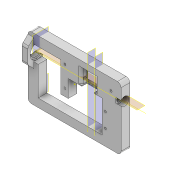
# Autodesk Inventor part: 10_Wellplate_base_v3
Saved by Autodesk Inventor 2022 (Build 260153000, 153)
## iProperties
Created: 2022-04-18
Part Number: 10_Wellplate_base_v3
Material: Generic
Document SubType Name: Modeling
Designer: Prakash Lab
Density: 1 g/cm^3
Appearance: Default
Author: Prakash Lab
Autodesk Inventor part; units mm, degrees
ref_plane "YZ Plane" through (0, 0, 0) normal (1, 0, 0) x (0, 1, 0)
ref_plane "XZ Plane" through (0, 0, 0) normal (0, 1, 0) x (-1, 0, 0)
ref_plane "XY Plane" through (0, 0, 0) normal (0, 0, 1) x (1, 0, 0)
sketch "Sketch1" plane through (0, 0, 0) normal (0, 0, 1) x (1, 0, 0)
  line L0 (63.9, -42.75) -> (-63.9, -42.75)
  line L1 (-63.9, -42.75) -> (-63.9, 42.75)
  line L2 (-63.9, 42.75) -> (63.9, 42.75)
  line L3 (63.9, 42.75) -> (63.9, -42.75)
  line L4 (63.9, -42.75) -> (-63.9, 42.75) construction
  line L5 (-63.9, -42.75) -> (63.9, 42.75) construction
  point P0 (0, 0)
  dimension "d0" = 127.8
  dimension "d1" = 85.5
  constraints: 12 end point, 2 midpoint, 2 parallel, 1 horizontal, 1 perpendicular
  measures "d0" distance of L0.start L0.end
  measures "d1" distance of L0.end L1.end
extrude "Extrusion1" add sketch "Sketch1" along normal blind 12
fillet "Fillet1" radius 4 4 edges at (63.9, 42.75, 6) (-63.9, 42.75, 6) (-63.9, -42.75, 6) (63.9, -42.75, 6)
sketch "Sketch2" plane through (0, 0, 12) normal (0, 0, 1) x (1, 0, 0)
  arc A0 (59.9, -42.75) -> (63.9, -38.75) centre (59.9, -38.75) ccw projected
  line L0 (63.9, -38.75) -> (63.9, 38.75) projected
  arc A1 (63.9, 38.75) -> (59.9, 42.75) centre (59.9, 38.75) ccw projected
  line L1 (59.9, 42.75) -> (-59.9, 42.75) projected
  arc A2 (-59.9, 42.75) -> (-63.9, 38.75) centre (-59.9, 38.75) ccw projected
  line L2 (-63.9, 38.75) -> (-63.9, -38.75) projected
  arc A3 (-63.9, -38.75) -> (-59.9, -42.75) centre (-59.9, -38.75) ccw projected
  line L3 (-59.9, -42.75) -> (59.9, -42.75) projected
  line L4 (28, 3) -> (9, 3)
  line L5 (9, 3) -> (9, 22)
  line L6 (9, 22) -> (28, 22)
  line L7 (28, 22) -> (28, 3)
  line L8 (28, 3) -> (9, 22) construction
  line L9 (9, 3) -> (28, 22) construction
  line L10 (18.6, 3.8849) -> (18.6, 4.1649)
  point P0 (0, 0)
  point P1 (18.5, 12.5)
  dimension "d5" = 19
  dimension "d6" = 19
  dimension "d221" = 3
  dimension "d223" = 18.5
  constraints: 14 end point, 2 midpoint, 2 parallel, 1 horizontal, 1 perpendicular, 1 vertical, 2 other
  measures "d5" distance of L5.end L6.end
  measures "d6" distance of L4.end L5.end
  measures "d221" vertical distance of L4.end point (0, 0)
  measures "d223" horizontal distance of point (0, 0) point (18.5, 12.5)
extrude "Extrusion2" cut sketch "Sketch2" against normal blind 8 contours L4 L5 L6 L7
sketch "Sketch3" plane through (0, 0, 4) normal (0, 0, 1) x (1, 0, 0)
  line L0 (9, 22) -> (28, 22) projected
  line L1 (9, 3) -> (9, 22) projected
  line L2 (28, 3) -> (9, 3) projected
  line L3 (28, 22) -> (28, 3) projected
  line L4 (26.5, 20.5) -> (10.5, 20.5)
  line L5 (10.5, 20.5) -> (10.5, 4.5)
  line L6 (10.5, 4.5) -> (26.5, 4.5)
  line L7 (26.5, 4.5) -> (26.5, 20.5)
  point P0 (0, 0)
  dimension "d11" = 1.5
  constraints: 8 end point, 3 other
  measures "d11" distance between parallel lines of L0 L4
extrude "Extrusion3" cut sketch "Sketch3" against normal through all contours L7 L6 L5 L4
ref_plane "Work Plane1" through (18.5, 3, 12) normal (-1, 0, 0) x (0, 0, 1)
ref_plane "Work Plane2" through (9, 12.5, 12) normal (0, 1, 0) x (1, 0, 0)
chamfer "Chamfer1" distance 4 angle 45 4 edges at (18.5, 4.5, 0) (26.5, 12.5, 0) (18.5, 20.5, 0) (10.5, 12.5, 0)
ref_plane "Work Plane3" through (28.5, 3, 12) normal (-1, 0, 0) x (0, 0, 1)
sketch "Sketch12" plane through (63.9, -38.75, 0) normal (1, 0, 0) x (0, 0, -1)
  circle A0 centre (-7.125, 48) radius 4.2 construction
  circle A1 centre (-7.125, 48) radius 4.5
  point P0 (0, 38.75)
  dimension "d100" = 9
  constraints: 1 centre point
  measures "d100" diameter of A1
extrude "Extrusion12" cut sketch "Sketch12" against normal up to surface (35.9 mm away) draft -4
sketch "Sketch13" plane through (63.9, -38.75, 0) normal (1, 0, 0) x (0, 0, -1)
  arc A0 (-10, 44.9382) -> (-10, 51.0618) centre (-7.125, 48) ccw projected
  circle A1 centre (-7.125, 48) radius 6
  point P0 (0, 38.75)
  dimension "d63" = 12
  constraints: 1 centre point, 1 coincident
  measures "d63" diameter of A1
extrude "Extrusion13" cut sketch "Sketch13" against normal blind 7
mirror "Mirror1" about plane through (18.5, 3, 12) normal (-1, 0, 0) of "Extrusion12", "Extrusion13"
ref_plane "Work Plane4" through (-47.9, 27.75, 11) normal (-1, 0, 0) x (0, 0, 1)
ref_plane "Work Plane5" through (-39.7, 19.25, 21) normal (0, 0, 1) x (1, 0, 0)
ref_plane "Arbeitsebene7" through (-58.9, -38.75, 0) normal (-1, 0, 0) x (0, 0, 1)
sketch "Skizze28" plane through (-58.9, -38.75, 0) normal (-1, 0, 0) x (0, 0, 1)
  line L0 (17.125, 56.5) -> (17.125, 39.5) projected
  arc A0 (17.125, 56.5) -> (15.625, 58) centre (15.625, 56.5) ccw projected
  line L1 (-1.375, 58) -> (15.625, 58) projected
  arc A1 (-1.375, 58) -> (-2.875, 56.5) centre (-1.375, 56.5) ccw projected
  line L2 (-2.875, 39.5) -> (-2.875, 56.5) projected
  arc A2 (-2.875, 39.5) -> (-1.375, 38) centre (-1.375, 39.5) ccw projected
  line L3 (15.625, 38) -> (-1.375, 38) projected
  arc A3 (15.625, 38) -> (17.125, 39.5) centre (15.625, 39.5) ccw projected
  circle A4 centre (15.125, 56) radius 0.7835 projected
  circle A5 centre (15.125, 40) radius 0.7835 projected
  circle A6 centre (-0.875, 56) radius 0.7835 projected
  circle A7 centre (-0.875, 40) radius 0.7835 projected
  circle A8 centre (7.125, 48) radius 7.5 projected
  arc A9 (17.625, 56.5) -> (15.625, 58.5) centre (15.625, 56.5) ccw
  line L4 (17.625, 56.5) -> (17.625, 39.5)
  arc A10 (15.625, 37.5) -> (17.625, 39.5) centre (15.625, 39.5) ccw
  line L5 (15.625, 37.5) -> (-1.375, 37.5)
  arc A11 (-3.375, 39.5) -> (-1.375, 37.5) centre (-1.375, 39.5) ccw
  line L6 (-3.375, 39.5) -> (-3.375, 56.5)
  arc A12 (-1.375, 58.5) -> (-3.375, 56.5) centre (-1.375, 56.5) ccw
  line L7 (-1.375, 58.5) -> (15.625, 58.5)
  point P0 (0, 38.75)
  dimension "d142" = 0.5
  constraints: 8 end point, 8 point on circle, 4 centre point, 7 other
  measures "d142" distance between parallel lines of L1 L7
extrude "Extrusion27" cut sketch "Skizze28" against normal blind 40 contours L0 A3 L3 A2 L2 A1 L1 A0 | A4 | A5 | A6 | A7 | A8 | L4 A10 L5 A11 L6 A12 L7 A9
sketch "Skizze29" plane through (-63.9, -38.75, 0) normal (-1, 0, 0) x (0, 0, 1)
  line L0 (17.125, 56.5) -> (17.125, 39.5) projected
  arc A0 (17.125, 56.5) -> (15.625, 58) centre (15.625, 56.5) ccw projected
  line L1 (-1.375, 58) -> (15.625, 58) projected
  arc A1 (-1.375, 58) -> (-2.875, 56.5) centre (-1.375, 56.5) ccw projected
  line L2 (-2.875, 39.5) -> (-2.875, 56.5) projected
  arc A2 (-2.875, 39.5) -> (-1.375, 38) centre (-1.375, 39.5) ccw projected
  line L3 (15.625, 38) -> (-1.375, 38) projected
  arc A3 (15.625, 38) -> (17.125, 39.5) centre (15.625, 39.5) ccw projected
  circle A4 centre (15.125, 56) radius 0.7835 projected
  circle A5 centre (15.125, 40) radius 0.7835 projected
  circle A6 centre (-0.875, 56) radius 0.7835 projected
  circle A7 centre (-0.875, 40) radius 0.7835 projected
  circle A8 centre (7.125, 48) radius 7.5 projected
  line L4 (0, 77.5) -> (0, 0) projected
  line L5 (12, 77.5) -> (12, 0) projected
  line L6 (12, 0) -> (12, 44.5022) projected
  line L7 (12, 29.511) -> (18.807, 36.318)
  line L8 (18.807, 59.682) -> (10, 68.489)
  line L9 (10, 68.5) -> (10, 31.5) projected
  line L10 (20.125, 39.5) -> (20.125, 56.5)
  arc A9 (20.125, 56.5) -> (15.625, 61) centre (15.625, 56.5) ccw
  line L11 (15.625, 61) -> (-1.375, 61)
  arc A10 (-1.375, 61) -> (-5.875, 56.5) centre (-1.375, 56.5) ccw
  line L12 (-5.875, 56.5) -> (-5.875, 39.5)
  arc A11 (-5.875, 39.5) -> (-1.375, 35) centre (-1.375, 39.5) ccw
  line L13 (-1.375, 35) -> (15.625, 35)
  arc A12 (15.625, 35) -> (20.125, 39.5) centre (15.625, 39.5) ccw
  point P0 (0, 38.75)
  point P1 (0, 58)
  point P2 (0, 38)
  point P3 (10, 11.9077)
  point P4 (10, 31.5)
  point P5 (12, 38)
  point P6 (12, 66.489)
  point P7 (12, 58)
  point P8 (10, 10.3787)
  point P9 (0, 45.6581)
  point P10 (0, 50.3419)
  dimension "d151" = 45
  dimension "d152" = 45
  dimension "d224" = 3
  constraints: 12 end point, 10 point on circle, 4 centre point, 1 tangent, 12 other
  measures "d151" angle of L1 L8
  measures "d152" angle of L3 L7
  measures "d224" distance between parallel lines of L0 L10
extrude "Extrusion28" add sketch "Skizze29" against normal blind 8 contours A0 L1 L5 L11 A9 L10 A12 L13 L3 A3 L0 | L0 A3 L3 L5 A8 L1 A0 | L5 A8 L9 L1 | L3 L9 A8 L5 | L9 A8 L4 L1 | L5 L8 A9 L11 | L3 L4 A8 L9 | L13 A12 L7 L5 | L4 A8 | A4 | A5
sketch "Skizze30" plane through (-55.9, -38.75, 0) normal (1, 0, 0) x (0, 0, -1)
  circle A0 centre (-7.125, 48) radius 7.3 projected
  circle A1 centre (-7.125, 48) radius 7.8
  point P0 (0, 38.75)
  dimension "d147" = 0.5
  constraints: 1 centre point
  measures "d147" radial gap between concentric circles of A0 A1
extrude "Extrusion29" cut sketch "Skizze30" against normal up to surface (8 mm away) contours A0 | A1
fillet "Rundung6" radius 2 2 edges at (-59.9, 6.076, 0) (-59.9, 12.424, 0)
sketch "Skizze40" plane through (0, 0, 12) normal (0, 0, 1) x (1, 0, 0)
  line L0 (-63.9, -9.239) -> (-63.9, -38.75) projected
  arc A0 (-63.9, -38.75) -> (-59.9, -42.75) centre (-59.9, -38.75) ccw projected
  line L1 (-59.9, -42.75) -> (59.9, -42.75) projected
  arc A1 (59.9, -42.75) -> (63.9, -38.75) centre (59.9, -38.75) ccw projected
  line L2 (63.9, -38.75) -> (63.9, 5.7522) projected
  line L3 (63.9, 5.7522) -> (56.9, 5.7522) projected
  line L4 (56.9, 5.7522) -> (56.9, 12.7478) projected
  line L5 (56.9, 12.7478) -> (63.9, 12.7478) projected
  line L6 (63.9, 12.7478) -> (63.9, 38.75) projected
  arc A2 (63.9, 38.75) -> (59.9, 42.75) centre (59.9, 38.75) ccw projected
  line L7 (59.9, 42.75) -> (-59.9, 42.75) projected
  arc A3 (-59.9, 42.75) -> (-63.9, 38.75) centre (-59.9, 38.75) ccw projected
  line L8 (-63.9, 38.75) -> (-63.9, 27.739) projected
  line L9 (-55.9, 19.75) -> (-18.9, 19.75) projected
  line L10 (-18.9, 19.75) -> (-18.9, -1.25) projected
  line L11 (-18.9, -1.25) -> (-55.9, -1.25) projected
  line L12 (63.9, 12.7478) -> (63.9, 38.75) projected
  line L13 (-63.9, 42.75) -> (63.9, 42.75)
  line L14 (63.9, 42.75) -> (63.9, 32.75)
  line L15 (63.9, 32.75) -> (-63.9, 32.75)
  line L16 (-63.9, 32.75) -> (-63.9, 42.75)
  line L17 (-55.9, 27.739) -> (-55.9, 19.75) projected
  line L18 (-55.9, -1.25) -> (-55.9, -9.239) projected
  line L19 (-55.9, -9.239) -> (-63.9, -9.239) projected
  line L20 (-63.9, 27.739) -> (-55.9, 27.739) projected
  point P0 (0, 0)
  point P1 (-59.9, 42.75)
  dimension "d178" = 10
  constraints: 8 end point, 2 parallel, 1 horizontal, 1 perpendicular, 1 point on line
  measures "d178" distance of L13.end L14.end
extrude "Extrusion37" cut sketch "Skizze40" against normal through all contours L8 A3 L7 A2 L6 L15 | L16 L13 A3 | A2 L13 L14
sketch "Skizze41" plane through (0, 0, 12) normal (0, 0, 1) x (1, 0, 0)
  line L0 (63.9, 32.75) -> (-63.9, 32.75) projected
  line L1 (-63.9, 32.75) -> (-63.9, 27.739) projected
  line L2 (-55.9, 19.75) -> (-18.9, 19.75) projected
  line L3 (-18.9, 19.75) -> (-18.9, -1.25) projected
  line L4 (-18.9, -1.25) -> (-55.9, -1.25) projected
  line L5 (-63.9, -9.239) -> (-63.9, -38.75) projected
  arc A0 (-63.9, -38.75) -> (-59.9, -42.75) centre (-59.9, -38.75) ccw projected
  line L6 (-59.9, -42.75) -> (59.9, -42.75) projected
  arc A1 (59.9, -42.75) -> (63.9, -38.75) centre (59.9, -38.75) ccw projected
  line L7 (63.9, -38.75) -> (63.9, 5.7522) projected
  line L8 (63.9, 5.7522) -> (56.9, 5.7522) projected
  line L9 (56.9, 5.7522) -> (56.9, 12.7478) projected
  line L10 (56.9, 12.7478) -> (63.9, 12.7478) projected
  line L11 (63.9, 12.7478) -> (63.9, 32.75) projected
  line L12 (-63.9, -38.75) -> (63.9, -38.75)
  line L13 (63.9, -38.75) -> (63.9, -52.75)
  line L14 (63.9, -52.75) -> (-63.9, -52.75)
  line L15 (-63.9, -52.75) -> (-63.9, -38.75)
  line L16 (-63.9, 27.739) -> (-55.9, 27.739) projected
  line L17 (-55.9, 27.739) -> (-55.9, 19.75) projected
  line L18 (-55.9, -1.25) -> (-55.9, -9.239) projected
  line L19 (-55.9, -9.239) -> (-63.9, -9.239) projected
  point P0 (0, 0)
  dimension "d181" = 14
  constraints: 8 end point, 2 parallel, 1 horizontal, 1 perpendicular
  measures "d181" distance of L12.end L13.end
extrude "Extrusion38" add sketch "Skizze41" against normal up to surface (12 mm away) contours L13 L14 L15 A0 L6 A1
fillet "Rundung7" radius 5 4 edges at (-63.9, 32.75, 6) (63.9, 32.75, 6) (-63.9, -52.75, 6) (63.9, -52.75, 6)
sketch "Skizze42" plane through (0, 0, 12) normal (0, 0, 1) x (1, 0, 0)
  line L0 (34.4, -33.4236) -> (34.4, -16.1764)
  arc A0 (30.4, -33.4236) -> (34.4, -33.4236) centre (32.4, -33.4236) ccw
  line L1 (30.4, -16.1764) -> (30.4, -33.4236)
  arc A1 (34.4, -16.1764) -> (30.4, -16.1764) centre (32.4, -16.1764) ccw
  line L2 (25.4, -33.4236) -> (25.4, -21.25)
  arc A2 (25.4, -33.4236) -> (25.7804, -35.6997) centre (32.4, -33.4236) ccw
  arc A3 (23.8891, -38.35) -> (25.7804, -35.6997) centre (23.8891, -36.35) ccw
  line L3 (37.373, -38.35) -> (23.8891, -38.35)
  arc A4 (37.373, -38.35) -> (37.4, -38.3226) centre (32.4, -33.4236) ccw
  line L4 (37.4, -11.2774) -> (37.4, -38.3226)
  arc A5 (37.4, -11.2774) -> (37.373, -11.25) centre (32.4, -16.1764) ccw
  line L5 (27.427, -11.25) -> (37.373, -11.25)
  arc A6 (27.427, -11.25) -> (27.4, -11.2774) centre (32.4, -16.1764) ccw
  line L6 (27.4, -19.25) -> (27.4, -11.2774)
  arc A7 (25.4, -21.25) -> (27.4, -19.25) centre (25.4, -19.25) ccw
  arc A8 (12.0825, -21.5243) -> (11.6348, -21.331) centre (11.0716, -23.25) ccw
  spline S0 degree 3 poles (12.0825, -21.5243) (11.8555, -21.3913) (11.6488, -21.229) (11.2907, -20.8371) (11.1452, -20.6102) (10.9547, -20.1287) (10.906, -19.8824) (10.906, -19.633) knots 0 0 0 0 0.335568 0.335568 0.679419 0.679419 1 1 1 1
  line L7 (10.906, -11.25) -> (10.906, -19.633)
  line L8 (-7.9188, -11.25) -> (10.906, -11.25)
  arc A9 (-7.9188, -11.25) -> (-8.1, -11.4342) centre (-3.0199, -16.25) ccw
  line L9 (-8.1, -21.0658) -> (-8.1, -11.4342)
  arc A10 (-8.1, -21.0658) -> (-3.0199, -23.25) centre (-3.0199, -16.25) ccw
  line L10 (6.8199, -23.25) -> (-3.0199, -23.25)
  arc A11 (6.8199, -23.25) -> (11.6348, -21.331) centre (6.8199, -16.25) ccw
  arc A12 (-3.0199, -14.25) -> (-3.0199, -18.25) centre (-3.0199, -16.25) ccw
  line L11 (6.8199, -14.25) -> (-3.0199, -14.25)
  arc A13 (6.8199, -18.25) -> (6.8199, -14.25) centre (6.8199, -16.25) ccw
  line L12 (-3.0199, -18.25) -> (6.8199, -18.25)
  line L13 (11.7188, -21.25) -> (25.4, -21.25)
  arc A14 (6.8199, -23.25) -> (11.7188, -21.25) centre (6.8199, -16.25) ccw
  line L14 (6.8199, -23.25) -> (-3.0199, -23.25)
  arc A15 (-8.1, -21.0658) -> (-3.0199, -23.25) centre (-3.0199, -16.25) ccw
  line L15 (-8.1, -38.35) -> (-8.1, -21.0658)
  line L16 (2.9, -38.35) -> (-8.1, -38.35)
  line L17 (2.9, -32.85) -> (2.9, -38.35)
  line L18 (22.3, -32.85) -> (2.9, -32.85)
  line L19 (22.3, -32.85) -> (22.3, -38.35)
  line L20 (22.3, -38.35) -> (23.8891, -38.35)
  arc A16 (23.8891, -38.35) -> (25.7804, -35.6997) centre (23.8891, -36.35) ccw
  arc A17 (25.4, -33.4236) -> (25.7804, -35.6997) centre (32.4, -33.4236) ccw
  line L21 (25.4, -33.4236) -> (25.4, -21.25)
  circle A18 centre (6.8199, -6.25) radius 3.25
  circle A19 centre (32.4, -6.25) radius 3.25
  circle A20 centre (-3.0199, -6.25) radius 3.25
  line L22 (-18.1, -1.25) -> (47.4, -1.25)
  line L23 (-58.9, -52.75) -> (58.9, -52.75)
  line L24 (58.9, -52.75) -> (-58.9, -52.75)
  line L25 (7.9, -11.25) -> (27.427, -11.25)
  line L26 (47.4, -11.25) -> (47.4, -1.25)
  line L27 (-18.1, -1.25) -> (-18.1, -21.25)
  line L28 (-11.5, -4.75) -> (-11.5, -17.75)
  arc A21 (-14.7, -17.75) -> (-11.5, -17.75) centre (-13.1, -17.75) ccw
  line L29 (-14.7, -17.75) -> (-14.7, -4.75)
  arc A22 (-11.5, -4.75) -> (-14.7, -4.75) centre (-13.1, -4.75) ccw
  line L30 (43.973, -4.75) -> (43.973, -17.75)
  arc A23 (40.773, -17.75) -> (43.973, -17.75) centre (42.373, -17.75) ccw
  line L31 (40.773, -17.75) -> (40.773, -4.75)
  arc A24 (43.973, -4.75) -> (40.773, -4.75) centre (42.373, -4.75) ccw
  line L32 (47.373, -11.25) -> (47.4, -11.25)
  line L33 (27.4, -11.2774) -> (27.4, -21.25)
  line L34 (27.4, -21.25) -> (37.4, -21.25)
  line L35 (-18.1, -21.25) -> (7.9, -21.25)
  line L36 (7.9, -21.25) -> (7.9, -11.25)
  line L37 (40.7865, -37.3611) -> (40.7865, -24.3611)
  arc A25 (43.9865, -24.3611) -> (40.7865, -24.3611) centre (42.3865, -24.3611) ccw
  line L38 (43.9865, -24.3611) -> (43.9865, -37.3611)
  arc A26 (40.7865, -37.3611) -> (43.9865, -37.3611) centre (42.3865, -37.3611) ccw
  line L39 (37.4, -21.25) -> (37.4, -41.25)
  line L40 (37.4, -41.25) -> (47.373, -41.25)
  line L41 (47.373, -41.25) -> (47.373, -11.25)
  line L42 (-58.9, -1.25) -> (-18.9, -1.25)
  line L43 (-49.9, -1.25) -> (-8.6, -1.25)
  line L44 (-8.6, -1.25) -> (-8.6, -41.35)
  line L45 (-8.6, -41.35) -> (-49.9, -41.35)
  line L46 (-49.9, -41.35) -> (-49.9, -1.25)
  line L47 (-63.9, -9.239) -> (-63.9, -47.75)
  line L48 (26.5, 4.5) -> (10.5, 4.5)
  line L49 (-8.6, 3.5) -> (37.9, 3.5)
  line L50 (37.9, 3.5) -> (37.9, -41.35)
  line L51 (37.9, -41.35) -> (-8.6, -41.35)
  line L52 (-8.6, -41.35) -> (-8.6, 3.5)
  circle A27 centre (-13.1, -11.2637) radius 1.4
  circle A28 centre (42.4, -11.2637) radius 1.4
  circle A29 centre (42.4, -31.25) radius 1.4
  line L53 (-18.9, 19.75) -> (-18.9, -1.25)
  line L54 (-18.1, -1.25) -> (-18.9, -1.25)
  line L55 (-18.9, -1.25) -> (-18.9, -21.25)
  line L56 (-18.9, -21.25) -> (-18.1, -21.25)
  line L57 (-18.1, -21.25) -> (-18.1, -1.25)
  arc A30 (27.427, -11.25) -> (27.4, -11.2774) centre (32.4, -16.1764) ccw
  line L58 (-18.9, -21.25) -> (-8.6, -21.25)
  line L59 (-8.6, -21.25) -> (-8.6, -41.35)
  line L60 (-8.6, -41.35) -> (-18.9, -41.35)
  line L61 (-18.9, -41.35) -> (-18.9, -21.25)
  point P0 (37.4, -13.25)
  point P1 (47.373, -21.25)
  point P2 (-8.1, -21.25)
  point P3 (-8.6, -38.75)
  point P4 (-8.6, -21.25)
  point P5 (-18.9, 10.3274)
  point P6 (-8.6, -21.25)
  point P7 (-63.9, -0.75)
  dimension "d199" = 14
  dimension "d201" = 0.5
  dimension "d203" = 0.5
  dimension "d204" = 1
  dimension "d205" = 3
  dimension "d206" = 2.8
  dimension "d207" = 2.8
  dimension "d208" = 2.8
  constraints: 32 end point, 8 parallel, 4 horizontal, 4 perpendicular, 3 centre point, 2 point on line, 1 other
  measures "d199" distance between parallel lines of L47 L46
  measures "d201" distance from line of L9.end L52
  measures "d203" distance between parallel lines of L4 L50
  measures "d204" distance between parallel lines of L48 L49
  measures "d205" distance between parallel lines of L3 L51
  measures "d206" diameter of A27
  measures "d207" diameter of A28
  measures "d208" diameter of A29
extrude "Extrusion39" cut sketch "Skizze42" against normal through all contours A0 L1 L34 L0 | L0 L34 L4 A4 L3 A3 A2 L2 A7 L33 L1 A0 | L34 L1 A1 L0 | L0 A1 L1 L34 L33 L6 A6 L5 A5 L4 | L4 A5 L5 L25 L8 A9 L9 L15 L35 L44 L22 L50 L40 L39 | L39 L40 L50 L51 L44 L35 L15 L16 L17 L18 L19 L20 L3 A4 | A7 L13 A14 S0 L7 L25 A6 L6 | L2 A2 A3 L20 L19 L18 L17 L16 L15 L35 A10 L10 A11 A8 S0 A14 L13 | L7 S0 A14 A11 L10 A10 L35 L36 A13 L8 | L22 L52 L49 L50 | S0 A8 A14 | L36 A13 L11 A12 L12 L35 A10 L9 A9 L8 | L45 L61 L56 L35 L44 | L36 A13 L12 A12 L11 | A13 L36 | L45 L46 L42 L55 L61 | L15 A10 L35 | A18 | A19 | A20 | A27 | A28 | A29
sketch "Skizze44" plane through (0, 0, 12) normal (0, 0, 1) x (1, 0, 0)
  point P0 (0, 0)
sketch "Skizze45" plane through (-55.9, -38.75, 0) normal (1, 0, 0) x (0, 0, -1)
  arc A0 (-3.0459, 54.6484) -> (-3.0459, 41.3516) centre (-7.125, 48) ccw projected
  circle A1 centre (-7.125, 48) radius 10
  point P0 (0, 38.75)
  dimension "d195" = 20
  constraints: 1 centre point, 1 coincident
  measures "d195" diameter of A1
extrude "Extrusion41" cut sketch "Skizze45" against normal blind 2
sketch "Skizze46" plane through (0, 0, 12) normal (0, 0, 1) x (1, 0, 0)
  line L0 (-8.6, 3.5) -> (9, 3.5) projected
  line L1 (9, 3.5) -> (9, 22) projected
  line L2 (9, 22) -> (28, 22) projected
  line L3 (28, 22) -> (28, 3.5) projected
  line L4 (37.9, 3.5) -> (37.9, -41.35) projected
  line L5 (37.9, -41.35) -> (-49.9, -41.35) projected
  line L6 (-49.9, -41.35) -> (-49.9, -1.25) projected
  line L7 (-49.9, -1.25) -> (-55.9, -1.25) projected
  line L8 (-63.9, -9.239) -> (-63.9, -47.75) projected
  arc A0 (-63.9, -47.75) -> (-58.9, -52.75) centre (-58.9, -47.75) ccw projected
  line L9 (-58.9, -52.75) -> (58.9, -52.75) projected
  arc A1 (58.9, -52.75) -> (63.9, -47.75) centre (58.9, -47.75) ccw projected
  line L10 (63.9, -47.75) -> (63.9, 5.7522) projected
  line L11 (63.9, 5.7522) -> (56.9, 5.7522) projected
  line L12 (56.9, 5.7522) -> (56.9, 12.7478) projected
  line L13 (56.9, 12.7478) -> (63.9, 12.7478) projected
  line L14 (63.9, 12.7478) -> (63.9, 27.75) projected
  arc A2 (63.9, 27.75) -> (58.9, 32.75) centre (58.9, 27.75) ccw projected
  line L15 (58.9, 32.75) -> (-58.9, 32.75) projected
  arc A3 (-58.9, 32.75) -> (-63.9, 27.75) centre (-58.9, 27.75) ccw projected
  line L16 (-55.9, 19.75) -> (-18.9, 19.75) projected
  line L17 (-18.9, 19.75) -> (-18.9, -21.25) projected
  line L18 (-18.9, -21.25) -> (-8.6, -21.25) projected
  line L19 (-8.6, -21.25) -> (-8.6, 3.5) projected
  circle A4 centre (42.4, -31.25) radius 1.4 projected
  circle A5 centre (42.4, -11.2637) radius 1.4 projected
  circle A6 centre (-13.1, -11.2637) radius 1.4 projected
  circle A7 centre (-13.1, 17.25) radius 1.4
  circle A8 centre (50.2191, 17.25) radius 1.4
  line L20 (28, 3.5) -> (37.9, 3.5) projected
  line L21 (-55.9, -1.25) -> (-55.9, -9.239) projected
  line L22 (-55.9, -9.239) -> (-63.9, -9.239) projected
  line L23 (-63.9, 27.739) -> (-55.9, 27.739) projected
  line L24 (-55.9, 27.739) -> (-55.9, 19.75) projected
  line L25 (-63.9, 27.75) -> (-63.9, 27.739) projected
  point P0 (0, 0)
  dimension "d209" = 2.8
  dimension "d210" = 2.8
  constraints: 2 centre point
  measures "d209" diameter of A7
  measures "d210" diameter of A8
extrude "Extrusion42" cut sketch "Skizze46" against normal through all contours A7 | A8
sketch "Skizze49" plane through (0, 0, 0) normal (0, 0, -1) x (-1, 0, 0)
  line L0 (9.6, 5.25) -> (2.6, 5.25) projected
  line L1 (-26.5, 4.5) -> (-10.5, 4.5) projected
  line L2 (6.6, 5.45) -> (-43.4, 5.45) projected
  line L3 (-37.9, 2.25) -> (-37.9, 5.25) projected
  line L4 (-30.5, 24.5) -> (-30.5, 3.5) projected
  line L5 (8.6, 2.25) -> (9.6, 2.25) projected
  line L6 (-46.4, 2.25) -> (-37.9, 2.25)
  line L7 (-37.9, 2.25) -> (-37.9, 4.5)
  line L8 (-37.9, 4.5) -> (-46.4, 4.5)
  line L9 (-46.4, 4.5) -> (-46.4, 2.25)
  line L10 (8.6, 2.25) -> (9.6, 2.25) projected
  line L11 (-37.9, 4.5) -> (9.6, 4.5)
  line L12 (9.6, 4.5) -> (9.6, 2.25)
  line L13 (9.6, 2.25) -> (-37.9, 2.25)
  line L14 (-37.9, 2.25) -> (-37.9, 4.5)
  point P0 (0, 0)
  point P1 (8.6, 2.25)
  point P2 (-10.5, 4.5)
  point P3 (-42.4, 6.25)
  point P4 (-41.0667, 6.25)
  point P5 (-30.5, 3.5)
  constraints: 16 end point, 4 parallel, 2 horizontal, 2 perpendicular, 1 point on line, 1 other
ref_plane "Arbeitsebene10" through (-6.6, 5.45, 2.125) normal (0, 0, -1) x (0, 1, 0)
extrude "Extrusion45" add sketch "Skizze49" against normal up to surface (4 mm away) contours L3 L6 L9 L8
sketch "Skizze50" plane through (-8.6, 3.5, 12) normal (0, -1, 0) x (1, 0, 0)
  line L0 (17.6, 0) -> (36.6, 0) projected
  line L1 (17.6, 0) -> (17.6, -8) projected
  line L2 (17.6, -8) -> (36.6, -8) projected
  line L3 (36.6, 0) -> (36.6, -8) projected
  line L4 (17.6, 0) -> (36.6, 0) projected
  line L5 (18.6, 0) -> (35.6, 0)
  line L6 (35.6, 0) -> (35.6, -7)
  line L7 (35.6, -7) -> (18.6, -7)
  line L8 (18.6, -7) -> (18.6, 0)
  line L9 (19.1, -8) -> (15.1, -12) projected
  line L10 (35.1, -8) -> (39.1, -12) projected
  line L11 (36.1, -9) -> (18.1, -9) projected
  line L12 (18.1, -9) -> (19.1, -8) projected
  line L13 (35.1, -8) -> (19.1, -8) projected
  line L14 (35.1, -8) -> (36.1, -9) projected
  line L15 (15.1, -12) -> (39.1, -12) projected
  line L16 (15.1, -12) -> (-0.7627, -12)
  line L17 (-50.3, -12) -> (67.5, -12) projected
  line L18 (-0.7627, 0) -> (-0.7627, -12)
  line L19 (-0.7627, 0) -> (17.6, 0)
  line L20 (36.6, 0) -> (36.6, -8) projected
  line L21 (36.6, 0) -> (47.1, 0)
  line L22 (47.1, 0) -> (47.1, -12)
  line L23 (47.1, -12) -> (39.1, -12)
  point P0 (8.6, -12)
  point P1 (35.6, 0)
  point P2 (35.6, -8)
  point P3 (35.6, 0)
  dimension "d225" = 1
  dimension "d226" = 1
  dimension "d229" = 1
  constraints: 21 end point, 5 perpendicular, 4 point on line, 2 parallel, 1 horizontal
  measures "d225" distance between parallel lines of L1 L8
  measures "d226" distance between parallel lines of L3 L6
  measures "d229" distance between parallel lines of L2 L7
extrude "Extrusion46" add sketch "Skizze50" along normal blind 1 contours L0 L8 L7 L6 L3 L2 L1 | L1 L2 L9 L16 L18 L19 | L2 L10 L11 L9 | L21 L22 L17 L10 L2 L3 | L11 L10 L15 L9
chamfer "Fase3" distance 3 angle 45 3 edges at (18.5, 22, 12) (9, 12.75, 12) (28, 12.75, 12)
body "Solid1"
